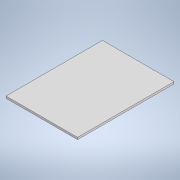
# Autodesk Inventor part: plate2
Saved by Autodesk Inventor 2020 (Build 240168000, 168)
## iProperties
Created: 2020-07-26
Part Number: plate2
Material: Generic
Document SubType Name: Modeling
Designer: Aarya
Density: 1 g/cm^3
Appearance: Default
Author: Aarya
Autodesk Inventor part; units mm, degrees
ref_plane "YZ Plane" through (0, 0, 0) normal (1, 0, 0) x (0, 1, 0)
ref_plane "XZ Plane" through (0, 0, 0) normal (0, 1, 0) x (-1, 0, 0)
ref_plane "XY Plane" through (0, 0, 0) normal (0, 0, 1) x (1, 0, 0)
sketch "Sketch1" plane through (0, 0, 0) normal (0, 1, 0) x (-1, 0, 0)
  line L0 (36.1015, 48.6655) -> (-36.1015, 48.6655)
  line L1 (-36.1015, 48.6655) -> (-36.1015, -48.6655)
  line L2 (-36.1015, -48.6655) -> (36.1015, -48.6655)
  line L3 (36.1015, -48.6655) -> (36.1015, 48.6655)
  line L4 (36.1015, 48.6655) -> (-36.1015, -48.6655) construction
  line L5 (-36.1015, 48.6655) -> (36.1015, -48.6655) construction
  point P0 (0, 0)
  dimension "d0" = 97.331
  dimension "d1" = 72.203
  constraints: 12 end point, 2 midpoint, 2 parallel, 1 horizontal, 1 perpendicular
  measures "d0" distance of L2.end L0.start
  measures "d1" distance of L0.start L0.end
extrude "Extrusion1" add sketch "Sketch1" along normal blind 2
body "Solid1"
